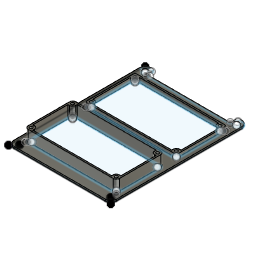
uconsole-shell-back-seprate-part-a-final (Autodesk Fusion 360 design; units mm, degrees)
Autodesk Fusion 360 part; units mm, degrees
note: some values were not read from the file. Set by a fixed rule: which sketch regions a step uses.
sketch "草图1" plane through (0, 0, 0) normal (0, 0, 1) x (1, 0, 0)
  line L0 (7, 0) -> (124, 0)
  line L1 (131, 7) -> (131, 168)
  line L2 (0, 168) -> (0, 7)
  line L3 (14, 165) -> (117, 165)
  line L4 (12, 167) -> (12, 173)
  line L5 (119, 167) -> (119, 173)
  arc A0 (7, 175) -> (0, 168) centre (7, 168) ccw
  arc A1 (131, 168) -> (124, 175) centre (124, 168) ccw
  circle A2 centre (7, 168) radius 2
  circle A3 centre (7, 168) radius 2.5
  circle A4 centre (7, 168) radius 3.7
  circle A5 centre (124, 168) radius 2
  circle A6 centre (124, 168) radius 2.5
  circle A7 centre (124, 168) radius 3.7
  line L6 (7, 175) -> (10, 175)
  line L7 (121, 175) -> (124, 175)
  arc A8 (121, 175) -> (119, 173) centre (121, 173) ccw
  arc A9 (117, 165) -> (119, 167) centre (117, 167) ccw
  arc A10 (12, 173) -> (10, 175) centre (10, 173) ccw
  arc A11 (12, 167) -> (14, 165) centre (14, 167) ccw
  arc A12 (0, 7) -> (7, 0) centre (7, 7) ccw
  arc A13 (124, 0) -> (131, 7) centre (124, 7) ccw
  circle A14 centre (7, 7) radius 2
  circle A15 centre (7, 7) radius 2.5
  circle A16 centre (7, 7) radius 3.7
  circle A17 centre (124, 7) radius 2
  circle A18 centre (124, 7) radius 2.5
  circle A19 centre (124, 7) radius 3.7
  line L8 (11, 14.0612) -> (120, 14.0612)
  line L9 (124, 18.0612) -> (124, 71.0612)
  line L10 (120, 75.0612) -> (11, 75.0612)
  line L11 (7, 71.0612) -> (7, 18.0612)
  line L12 (12, 16) -> (119, 16)
  line L13 (122, 19) -> (122, 70)
  line L14 (119, 73) -> (12, 73)
  line L15 (9, 70) -> (9, 19)
  arc A20 (11, 75.0612) -> (7, 71.0612) centre (11, 71.0612) ccw
  arc A21 (12, 73) -> (9, 70) centre (12, 70) ccw
  arc A22 (124, 71.0612) -> (120, 75.0612) centre (120, 71.0612) ccw
  arc A23 (122, 70) -> (119, 73) centre (119, 70) ccw
  arc A24 (7, 18.0612) -> (11, 14.0612) centre (11, 18.0612) ccw
  arc A25 (9, 19) -> (12, 16) centre (12, 19) ccw
  arc A26 (120, 14.0612) -> (124, 18.0612) centre (120, 18.0612) ccw
  arc A27 (119, 16) -> (122, 19) centre (119, 19) ccw
  line L16 (9, 155) -> (122, 155)
  line L17 (124, 153) -> (124, 93)
  line L18 (122, 91) -> (9, 91)
  line L19 (7, 93) -> (7, 153)
  line L20 (10, 153) -> (121, 153)
  line L21 (122, 152) -> (122, 94)
  line L22 (121, 93) -> (10, 93)
  line L23 (9, 94) -> (9, 152)
  arc A28 (9, 155) -> (7, 153) centre (9, 153) ccw
  arc A29 (124, 153) -> (122, 155) centre (122, 153) ccw
  arc A30 (7, 93) -> (9, 91) centre (9, 93) ccw
  arc A31 (122, 91) -> (124, 93) centre (122, 93) ccw
  arc A32 (10, 153) -> (9, 152) centre (10, 152) ccw
  arc A33 (9, 94) -> (10, 93) centre (10, 94) ccw
  arc A34 (122, 152) -> (121, 153) centre (121, 152) ccw
  arc A35 (121, 93) -> (122, 94) centre (121, 94) ccw
  circle A36 centre (11, 151) radius 1.9
  line L24 (15, 151) -> (15, 153)
  line L25 (11, 147) -> (9, 147)
  circle A37 centre (11, 95) radius 1.9
  line L26 (11, 99) -> (9, 99)
  line L27 (15, 93) -> (15, 95)
  circle A38 centre (120, 95) radius 1.9
  line L28 (116, 95) -> (116, 93)
  line L29 (120, 99) -> (122, 99)
  circle A39 centre (120, 151) radius 1.9
  line L30 (116, 151) -> (116, 153)
  line L31 (120, 147) -> (122, 147)
  circle A40 centre (11, 71) radius 1.9
  line L32 (15, 71) -> (15, 73)
  line L33 (11, 67) -> (9, 67)
  arc A41 (11, 67) -> (15, 71) centre (11, 71) ccw
  circle A42 centre (11, 18) radius 1.9
  line L34 (11, 22) -> (9, 22)
  line L35 (15, 16) -> (15, 18)
  arc A43 (15, 18) -> (11, 22) centre (11, 18) ccw
  arc A44 (15, 95) -> (11, 99) centre (11, 95) ccw
  arc A45 (11, 147) -> (15, 151) centre (11, 151) ccw
  arc A46 (116, 151) -> (120, 147) centre (120, 151) ccw
  arc A47 (120, 99) -> (116, 95) centre (120, 95) ccw
  circle A48 centre (120, 18) radius 1.9
  line L36 (116, 18) -> (116, 16)
  line L37 (120, 22) -> (122, 22)
  arc A49 (120, 22) -> (116, 18) centre (120, 18) ccw
  circle A50 centre (120, 70.9999) radius 1.9
  line L38 (116, 71) -> (116, 73)
  line L39 (120, 67) -> (122, 67)
  arc A51 (116, 71) -> (120, 67) centre (120, 71) ccw
  point P0 (131, 0)
  point P1 (0, 175)
  point P2 (12, 165)
  point P3 (119, 165)
  point P4 (7, 14.0612)
  point P5 (124, 14.0612)
  point P6 (7, 75.0612)
  point P7 (9, 16)
  point P8 (122, 16)
  point P9 (9, 73)
  point P10 (7, 155)
  point P11 (124, 155)
  point P12 (7, 91)
  point P13 (9, 153)
  point P14 (122, 153)
  point P15 (9, 93)
  dimension "d1" = 131
  dimension "d2" = 175
  dimension "d3" = 107
  dimension "d4" = 7
  dimension "d5" = 7
  dimension "d6" = 4
  dimension "d7" = 5
  dimension "d8" = 7.4
  dimension "d9" = 4
  dimension "d10" = 5
  dimension "d11" = 7.4
  dimension "d12" = 2
  dimension "d13" = 2
  dimension "d14" = 2
  dimension "d15" = 2
  dimension "d16" = 7
  dimension "d17" = 7
  dimension "d18" = 4
  dimension "d19" = 5
  dimension "d20" = 7.4
  dimension "d21" = 4
  dimension "d22" = 5
  dimension "d23" = 7.4
  dimension "d24" = 117
  dimension "d25" = 61
  dimension "d26" = 113
  dimension "d27" = 57
  dimension "d28" = 4
  dimension "d29" = 3
  dimension "d30" = 4
  dimension "d31" = 3
  dimension "d32" = 4
  dimension "d33" = 3
  dimension "d34" = 4
  dimension "d35" = 3
  dimension "d36" = 117
  dimension "d37" = 64
  dimension "d38" = 113
  dimension "d39" = 60
  dimension "d40" = 2
  dimension "d41" = 2
  dimension "d42" = 2
  dimension "d43" = 2
  dimension "d44" = 1
  dimension "d45" = 1
  dimension "d46" = 1
  dimension "d47" = 1
  dimension "d57" = 3.8
  dimension "d58" = 3.8
  dimension "d59" = 3.8
  dimension "d60" = 3.8
  dimension "d62" = 3.8
  dimension "d63" = 4
  dimension "d64" = 3.8
  dimension "d65" = 4
  dimension "d66" = 4
  dimension "d68" = 4
  dimension "d69" = 4
  dimension "d70" = 3.8
  dimension "d71" = 4
  dimension "d72" = 3.8
  dimension "d73" = 4
  constraint horizontal L0
  constraint vertical L1
  constraint vertical L2
  constraint horizontal L3
  constraint coincident P1 L2
  constraint tangent L2 A0
  constraint tangent L1 A1
  constraint concentric A0 A2
  constraint concentric A0 A3
  constraint concentric A2 A4
  constraint concentric A1 A5
  constraint concentric A1 A6
  constraint concentric A6 A7
  constraint tangent A0 L6
  constraint tangent A1 L7
  constraint tangent L5 A8
  constraint tangent L7 A8
  constraint coincident P3 L3
  constraint coincident P3 L5
  constraint tangent L3 A9
  constraint tangent L5 A9
  constraint tangent L4 A10
  constraint tangent L6 A10
  constraint coincident P2 L3
  constraint coincident P2 L4
  constraint tangent L3 A11
  constraint tangent L4 A11
  constraint coincident origin L0
  constraint coincident origin L2
  constraint tangent L0 A12
  constraint tangent L2 A12
  constraint coincident P0 L0
  constraint coincident P0 L1
  constraint tangent L0 A13
  constraint tangent L1 A13
  constraint concentric A12 A14
  constraint concentric A12 A15
  constraint concentric A15 A16
  constraint concentric A13 A17
  constraint concentric A17 A18
  constraint concentric A17 A19
  constraint horizontal L8
  constraint vertical L9
  constraint horizontal L10
  constraint vertical L11
  constraint horizontal L12
  constraint vertical L13
  constraint horizontal L14
  constraint vertical L15
  constraint coincident P6 L10
  constraint coincident P6 L11
  constraint tangent L10 A20
  constraint tangent L11 A20
  constraint coincident P9 L14
  constraint coincident P9 L15
  constraint tangent L14 A21
  constraint tangent L15 A21
  constraint tangent L9 A22
  constraint tangent L10 A22
  constraint tangent L13 A23
  constraint tangent L14 A23
  constraint coincident P4 L8
  constraint coincident P4 L11
  constraint tangent L8 A24
  constraint tangent L11 A24
  constraint coincident P7 L12
  constraint coincident P7 L15
  constraint tangent L12 A25
  constraint tangent L15 A25
  constraint coincident P5 L8
  constraint coincident P5 L9
  constraint tangent L8 A26
  constraint tangent L9 A26
  constraint coincident P8 L12
  constraint coincident P8 L13
  constraint tangent L12 A27
  constraint tangent L13 A27
  constraint horizontal L16
  constraint vertical L17
  constraint horizontal L18
  constraint vertical L19
  constraint horizontal L20
  constraint vertical L21
  constraint horizontal L22
  constraint vertical L23
  constraint coincident P10 L16
  constraint coincident P10 L19
  constraint tangent L16 A28
  constraint tangent L19 A28
  constraint coincident P11 L16
  constraint coincident P11 L17
  constraint tangent L16 A29
  constraint tangent L17 A29
  constraint coincident P12 L18
  constraint coincident P12 L19
  constraint tangent L18 A30
  constraint tangent L19 A30
  constraint tangent L17 A31
  constraint tangent L18 A31
  constraint coincident P13 L20
  constraint coincident P13 L23
  constraint tangent L20 A32
  constraint tangent L23 A32
  constraint coincident P15 L22
  constraint coincident P15 L23
  constraint tangent L22 A33
  constraint tangent L23 A33
  constraint coincident P14 L20
  constraint coincident P14 L21
  constraint tangent L20 A34
  constraint tangent L21 A34
  constraint tangent L21 A35
  constraint tangent L22 A35
  constraint coincident L20 L24.end
  constraint perpendicular L20 L24
  constraint coincident L23 L25.end
  constraint perpendicular L23 L25
  constraint coincident L23 L26.end
  constraint perpendicular L23 L26
  constraint coincident L22 L27.start
  constraint perpendicular L22 L27
  constraint coincident L22 L28.end
  constraint perpendicular L22 L28
  constraint coincident L21 L29.end
  constraint perpendicular L21 L29
  constraint coincident L20 L30.end
  constraint perpendicular L20 L30
  constraint coincident L21 L31.end
  constraint perpendicular L21 L31
  constraint coincident L14 L32.end
  constraint perpendicular L14 L32
  constraint coincident L15 L33.end
  constraint perpendicular L15 L33
  constraint tangent L32 A41
  constraint tangent L33 A41
  constraint coincident L15 L34.end
  constraint perpendicular L15 L34
  constraint coincident L12 L35.start
  constraint perpendicular L12 L35
  constraint tangent L34 A43
  constraint tangent L35 A43
  constraint tangent L26 A44
  constraint tangent L27 A44
  constraint tangent L24 A45
  constraint tangent L25 A45
  constraint tangent L30 A46
  constraint tangent L31 A46
  constraint tangent L28 A47
  constraint tangent L29 A47
  constraint coincident L12 L36.end
  constraint perpendicular L12 L36
  constraint coincident L13 L37.end
  constraint perpendicular L13 L37
  constraint tangent L36 A49
  constraint tangent L37 A49
  constraint coincident L14 L38.end
  constraint perpendicular L14 L38
  constraint coincident L13 L39.end
  constraint perpendicular L13 L39
  constraint tangent L38 A51
  constraint tangent L39 A51
  measures "d1" distance of origin P0
  measures "d2" distance of origin P1
  measures "d3" distance of P2 P3
  measures "d4" radius of A0
  measures "d5" radius of A1
  measures "d6" diameter of A2
  measures "d7" diameter of A3
  measures "d8" diameter of A4
  measures "d9" diameter of A5
  measures "d10" diameter of A6
  measures "d11" diameter of A7
  measures "d12" radius of A8
  measures "d13" radius of A9
  measures "d14" radius of A10
  measures "d15" radius of A11
  measures "d16" radius of A12
  measures "d17" radius of A13
  measures "d18" diameter of A14
  measures "d19" diameter of A15
  measures "d20" diameter of A16
  measures "d21" diameter of A17
  measures "d22" diameter of A18
  measures "d23" diameter of A19
  measures "d24" distance of P4 P5
  measures "d25" distance of P4 P6
  measures "d26" distance of P7 P8
  measures "d27" distance of P7 P9
  measures "d28" radius of A20
  measures "d29" radius of A21
  measures "d30" radius of A22
  measures "d31" radius of A23
  measures "d32" radius of A24
  measures "d33" radius of A25
  measures "d34" radius of A26
  measures "d35" radius of A27
  measures "d36" distance of P10 P11
  measures "d37" distance of P10 P12
  measures "d38" distance of P13 P14
  measures "d39" distance of P13 P15
  measures "d40" radius of A28
  measures "d41" radius of A29
  measures "d42" radius of A30
  measures "d43" radius of A31
  measures "d44" radius of A32
  measures "d45" radius of A33
  measures "d46" radius of A34
  measures "d47" radius of A35
  measures "d57" diameter of A36
  measures "d58" diameter of A37
  measures "d59" diameter of A38
  measures "d60" diameter of A39
  measures "d62" diameter of A40
  measures "d63" radius of A41
  measures "d64" diameter of A42
  measures "d65" radius of A43
  measures "d66" radius of A44
  measures "d68" radius of A46
  measures "d69" radius of A47
  measures "d70" diameter of A48
  measures "d71" radius of A49
  measures "d72" diameter of A50
  measures "d73" radius of A51
extrude "拉伸13" cut sketch "草图1" along normal blind 16 contours A25 A42 picked at (9.8084, 16.8084)
extrude "拉伸14" cut sketch "草图1" along normal blind 16 contours A21 A40 picked at (10.7309, 71.3245)
extrude "拉伸15" cut sketch "草图1" along normal blind 16 contours A23 A50 picked at (121.1681, 72.2139)
extrude "拉伸16" cut sketch "草图1" along normal blind 16 contours A27 A48 picked at (120.3296, 17.7354)
extrude "拉伸17" add sketch "草图1" along normal blind 2 separate body contours L0 L1 L2 L3 L4 L5 A0 A1 L6 L7 A8 A9 A10 A11 A12 A13 | A3 | A4 | A6 | A7 | A15 | A16 | A18 | A19
extrude "拉伸18" add sketch "草图1" along normal blind 6 contours L16 L17 L18 L19 A28 A29 A30 A31 | L20 L23 A32 L24 L25 A45 | L20 L21 A34 L30 L31 A46 | L22 L23 A33 L26 L27 A44 | L21 L22 A35 L28 L29 A47
extrude "拉伸19" add sketch "草图1" along normal blind 16 contours L8 L9 L10 L11 A20 A22 A24 A26 | L12 L15 A25 A42 L34 L35 A43 | L12 L13 A27 A48 L36 L37 A49 | L14 L15 A21 A40 L32 L33 A41 | L13 L14 A23 A50 L38 L39 A51
extrude "拉伸20" cut sketch "草图1" against normal blind 0.4 from surface at 2 contours A3
extrude "拉伸21" cut sketch "草图1" against normal blind 0.4 from surface at 2 contours A6
extrude "拉伸22" cut sketch "草图1" against normal blind 0.4 from surface at 2 contours A18
extrude "拉伸23" cut sketch "草图1" against normal blind 0.4 from surface at 2 contours A15
